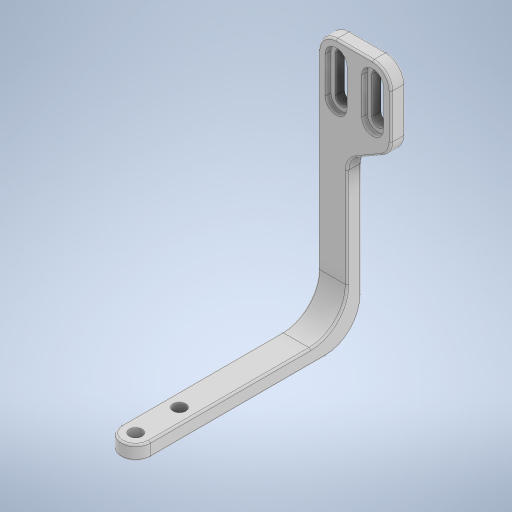
# Autodesk Inventor part: nozzlecleaner
Saved by Autodesk Inventor 2024.2 (Build 282272000, 272)
## iProperties
Created: 2024-07-30
Part Number: nozzlecleaner
Material: Generic
Document SubType Name: Modeling
Designer: Eric
Density: 1 g/cm^3
Appearance: Default
Author: Eric
Autodesk Inventor part; units mm, degrees
ref_plane "YZ Plane" through (0, 0, 0) normal (1, 0, 0) x (0, 1, 0)
ref_plane "XZ Plane" through (0, 0, 0) normal (0, 1, 0) x (-1, 0, 0)
ref_plane "XY Plane" through (0, 0, 0) normal (0, 0, 1) x (1, 0, 0)
sketch "Sketch1" plane through (0, 0, 0) normal (1, 0, 0) x (0, 1, 0)
  line L0 (0, 0) -> (0, -58)
  line L1 (0, -58) -> (67, -58)
  line L2 (67, -58) -> (67, -62)
  line L3 (67, -62) -> (-4, -62)
  line L4 (-4, -62) -> (-4, 0)
  line L5 (-4, 0) -> (0, 0)
  line L6 (57, -58) -> (57, -62) construction
  dimension "d0" = 10
  dimension "d2" = 57
  dimension "d3" = 62
  dimension "d4" = 4
  dimension "d5" = 4
  constraints: 14 end point, 6 perpendicular, 2 point on line, 1 vertical
  measures "d0" distance between parallel lines of L2 L6
  measures "d2" distance between parallel lines of L0 L6
  measures "d3" distance between parallel lines of L5 L3
  measures "d4" distance between parallel lines of L3 L1
  measures "d5" distance between parallel lines of L4 L0
extrude "Extrusion1" add sketch "Sketch1" along normal blind 8
fillet "Fillet1" radius 10 2 edges at (4, 0, -58) (4, -4, -62)
sketch "Sketch6" plane through (0, 67, -58) normal (0, 0, 1) x (1, 0, 0)
  line L0 (8, 0) -> (8, -57) projected
  line L1 (8, 0) -> (20, 0)
  line L2 (20, 0) -> (20, -20)
  line L3 (20, -20) -> (8, -26.9282)
  line L4 (0, 0) -> (0, -57) projected
  point P0 (0, -67)
  dimension "d31" = 20
  dimension "d32" = 20
  dimension "d33" = 60
  constraints: 6 end point, 1 horizontal, 1 perpendicular, 1 point on line
  measures "d31" distance between parallel lines of L4 L2
  measures "d32" distance from line of L1 L2.end
  measures "d33" angle of L0 L3
extrude "Extrusion5" add sketch "Sketch6" against normal up to surface (4 mm away)
sketch "Sketch3" plane through (0, 67, -58) normal (0, 0, 1) x (1, 0, 0)
  line L0 (5, -5) -> (5, -15) construction
  line L1 (2, -5) -> (2, -15)
  line L2 (8, -15) -> (8, -5)
  arc A0 (8, -5) -> (2, -5) centre (5, -5) ccw
  arc A1 (2, -15) -> (8, -15) centre (5, -15) ccw
  line L3 (15, -5) -> (15, -15) construction
  line L4 (12, -5) -> (12, -15)
  line L5 (18, -15) -> (18, -5)
  arc A2 (18, -5) -> (12, -5) centre (15, -5) ccw
  arc A3 (12, -15) -> (18, -15) centre (15, -15) ccw
  line L6 (0, 0) -> (8, 0) projected
  line L7 (0, 0) -> (20, 0) projected
  line L8 (10, 0) -> (10, -29.5179) construction
  point P0 (0, -67)
  point P1 (5, -10)
  point P2 (15, -10)
  dimension "d10" = 3
  dimension "d11" = 10
  dimension "d12" = 5
  dimension "d13" = 10
  constraints: 18 end point, 8 point on circle, 8 tangent, 5 parallel, 4 centre point, 3 midpoint, 1 equal radius, 1 horizontal alignment, 1 vertical, 1 other
  measures "d10" radius of A1
  measures "d11" distance between parallel lines of L3 L0
  measures "d12" distance from line of L6 L0.start
  measures "d13" distance of L0.start L0.end
extrude "Extrusion2" cut sketch "Sketch3" against normal blind 1.5
sketch "Sketch4" plane through (0, 67, -59.5) normal (0, 0, 1) x (1, 0, 0)
  arc A0 (2, -15) -> (8, -15) centre (5, -15) ccw projected
  line L0 (8, -5) -> (8, -15) projected
  arc A1 (8, -5) -> (2, -5) centre (5, -5) ccw projected
  arc A2 (12, -15) -> (18, -15) centre (15, -15) ccw projected
  arc A3 (18, -5) -> (12, -5) centre (15, -5) ccw projected
  line L1 (12, -15) -> (12, -5) projected
  line L2 (5, -5) -> (5, -15) construction
  line L3 (3.25, -5) -> (3.25, -15)
  line L4 (6.75, -15) -> (6.75, -5)
  arc A4 (6.75, -5) -> (3.25, -5) centre (5, -5) ccw
  arc A5 (3.25, -15) -> (6.75, -15) centre (5, -15) ccw
  line L5 (15, -5) -> (15, -15) construction
  line L6 (13.25, -5) -> (13.25, -15)
  line L7 (16.75, -15) -> (16.75, -5)
  arc A6 (16.75, -5) -> (13.25, -5) centre (15, -5) ccw
  arc A7 (13.25, -15) -> (16.75, -15) centre (15, -15) ccw
  line L8 (18, -5) -> (18, -15) projected
  line L9 (2, -15) -> (2, -5) projected
  point P0 (0, -67)
  point P1 (5, -10)
  point P2 (15, -10)
  dimension "d16" = 1.75
  dimension "d17" = 1.75
  constraints: 16 end point, 8 point on circle, 8 tangent, 4 centre point, 3 parallel, 2 midpoint, 1 vertical
  measures "d16" radius of A4
  measures "d17" radius of A6
extrude "Extrusion3" cut sketch "Sketch4" against normal through all contours A4 L4 A5 L3 | A6 L7 A7 L6
sketch "Sketch5" plane through (0, 0, 0) normal (0, 1, 0) x (1, 0, 0)
  circle A0 centre (4, 4) radius 1.75
  circle A1 centre (4, 16) radius 1.75
  line L0 (8, 48) -> (8, 0) projected
  line L1 (0, 0) -> (8, 0) projected
  line L2 (0, 48) -> (0, 0) projected
  dimension "d20" = 12
  dimension "d21" = 3.5
  dimension "d29" = 4
  dimension "d30" = 4
  constraints: 2 centre point, 1 equal radius, 1 point on line, 1 vertical alignment
  measures "d20" distance of A1.centre A0.centre
  measures "d21" diameter of A0
  measures "d29" distance from line of L1 A0.centre
  measures "d30" distance from line of L2 A0.centre
extrude "Extrusion4" cut sketch "Sketch5" against normal through all
fillet "Fillet2" radius 4 2 edges at (8, -2, 0) (0, -2, 0)
fillet "Fillet3" radius 5 4 edges at (20, 67, -60) (0, 67, -60) (8, 40.0718, -60) (20, 47, -60)
fillet "Fillet4" radius 0.5 32 edges at (6.8285, 0, -1.1715) (1.1715, 0, -1.1715) (4, 0, 0) (0, 0, -25.9999) (0, 2.9289, -55.0711) (0, 36, -58) (1.4645, 65.5355, -58) (10, 67, -58) (18.5355, 65.5355, -58) (20, 55.9434, -58) (19.3301, 47.3868, -58) (14, 43.5359, -58) (8.6699, 39.685, -58) (8, 23.5925, -58) (8, 2.9289, -55.0711) (8, 0, -25.9999) (8, -1.0711, -59.0711) (8, 21.5925, -62) (8.6699, 39.685, -62) (14, 43.5359, -62) (19.3301, 47.3868, -62) (20, 55.9434, -62) (18.5355, 65.5355, -62) (10, 67, -62) (1.4645, 65.5355, -62) (0, 34, -62) (0, -1.0711, -59.0711) (0, -4, -28) (1.1715, -4, -1.1715) (4, -4, 0) (6.8285, -4, -1.1715) (8, -4, -28)
sketch "Sketch7" plane through (4, -4, -4) normal (0, -1, 0) x (1, 0, 0)
  circle A0 centre (0, 0) radius 1.75 projected
  circle A1 centre (0, -12) radius 1.75 projected
  arc A2 (3.5, 0) -> (-3.5, 0) centre (0, 0) ccw projected
  line L0 (0, -3.2909) -> (-2.85, -1.6454)
  line L1 (-2.85, -1.6454) -> (-2.85, 1.6454)
  line L2 (-2.85, 1.6454) -> (0, 3.2909)
  line L3 (0, 3.2909) -> (2.85, 1.6454)
  line L4 (2.85, 1.6454) -> (2.85, -1.6454)
  line L5 (2.85, -1.6454) -> (0, -3.2909)
  line L6 (0, -15.2909) -> (-2.85, -13.6454)
  line L7 (-2.85, -13.6454) -> (-2.85, -10.3546)
  line L8 (-2.85, -10.3546) -> (0, -8.7091)
  line L9 (0, -8.7091) -> (2.85, -10.3546)
  line L10 (2.85, -10.3546) -> (2.85, -13.6454)
  line L11 (2.85, -13.6454) -> (0, -15.2909)
  point P0 (-4, 4)
  dimension "d39" = 5.7
  constraints: 24 end point, 2 coincident, 2 vertical, 1 collinear, 26 other
  measures "d39" distance between parallel lines of L1 L4
extrude "Extrusion6" cut sketch "Sketch7" against normal blind 1.5 contours A0 | A1 | L0 L1 L2 L3 L4 L5 | L6 L7 L8 L9 L10 L11
sketch "Sketch8" plane through (5, 66.5, -58) normal (0, 0, 1) x (1, 0, 0)
  point P0 (-5, -66.5)
body "Solid1"
